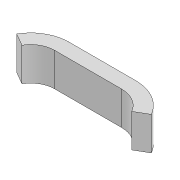
# Autodesk Inventor part: ArcSole2b
Saved by Autodesk Inventor 2022 (Build 260153000, 153)
## iProperties
Created: 2022-01-09
Part Number: ArcSole2b
Material: 一般
Document SubType Name: Modeling
Designer: tazak
Density: 1 g/cm^3
Appearance: 既定
Author: tazak
Autodesk Inventor part; units mm, degrees
ref_plane "YZ Plane" through (0, 0, 0) normal (1, 0, 0) x (0, 1, 0)
ref_plane "XZ Plane" through (0, 0, 0) normal (0, 1, 0) x (-1, 0, 0)
ref_plane "XY Plane" through (0, 0, 0) normal (0, 0, 1) x (1, 0, 0)
sketch "スケッチ1" plane through (0, 0, 0) normal (0, 1, 0) x (-1, 0, 0)
  circle A0 centre (70, -20) radius 80
  circle A1 centre (-70, -10) radius 90
  line L0 (70, -100) -> (-70, -100)
  line L1 (70, -20) -> (70, -100)
  line L2 (70, -20) -> (139.282, -60)
  line L3 (-70, -10) -> (-70, -100)
  line L4 (-70, -10) -> (-147.9423, -55)
  circle A2 centre (70, -20) radius 50
  circle A3 centre (-70, -10) radius 60
  line L5 (70, -70) -> (-70, -70)
  point P0 (0, 0)
  point P1 (113.3013, -45)
  point P2 (-121.9615, -40)
  dimension "d7" = 100
  dimension "d8" = 120
  dimension "d0" = 160
  dimension "d1" = 180
  dimension "d2" = 100
  dimension "d3" = 70
  dimension "d4" = 70
  dimension "d5" = 60
  dimension "d6" = 60
  constraints: 12 end point, 4 point on circle, 2 centre point, 2 coincident, 2 point on line, 2 tangent, 1 horizontal, 1 vertical, 6 other
  measures "d0" diameter of A0
  measures "d1" diameter of A1
  measures "d2" distance from line of L0 point (0, 0)
  measures "d3" horizontal distance of L0.start point (0, 0)
  measures "d4" horizontal distance of L0.end point (0, 0)
  measures "d5" angle of L1 L2
  measures "d6" angle of L4 L3
extrude "押し出し1" add sketch "スケッチ1" along normal mid plane 70 contours L1 A2 L2 A0 | L0 A1 L5 A0 | A0 L5 L1 | L3 L5 A1 | A1 L4 A3 L3
fillet "フィレット1" [suppressed]
